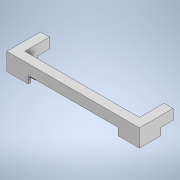
# Autodesk Inventor part: Glass ConnectorV2
Saved by Autodesk Inventor 2022 (Build 260153000, 153)
## iProperties
Created: 2022-05-30
Part Number: Glass ConnectorV2
Material: Generic
Document SubType Name: Modeling
Designer: abdoo
Density: 1 g/cm^3
Appearance: Default
Author: abdoo
Autodesk Inventor part; units mm, degrees
ref_plane "YZ Plane" through (0, 0, 0) normal (1, 0, 0) x (0, 1, 0)
ref_plane "XZ Plane" through (0, 0, 0) normal (0, 1, 0) x (-1, 0, 0)
ref_plane "XY Plane" through (0, 0, 0) normal (0, 0, 1) x (1, 0, 0)
sketch "Sketch1" plane through (0, 0, 0) normal (0, 1, 0) x (-1, 0, 0)
  line L0 (0, 0) -> (3.15, 0)
  line L1 (3.15, 0) -> (3.15, -20)
  line L2 (3.15, -20) -> (0, -20)
  line L3 (0, -20) -> (0, 0)
  line L4 (0, 0) -> (20, 0)
  line L5 (20, 0) -> (20, -3.15)
  line L6 (20, -3.15) -> (0, -3.15)
  line L7 (0, -3.15) -> (0, 0)
  line L8 (-1.5, 1.5) -> (4.65, 1.5)
  line L9 (4.65, 1.5) -> (4.65, -21.5)
  line L10 (4.65, -21.5) -> (-1.5, -21.5)
  line L11 (-1.5, -21.5) -> (-1.5, 1.5)
  line L12 (21.5, 1.5) -> (-1.5, 1.5)
  line L13 (-1.5, 1.5) -> (-1.5, -4.65)
  line L14 (-1.5, -4.65) -> (21.5, -4.65)
  line L15 (21.5, -4.65) -> (21.5, 1.5)
  line L16 (3.15, -20) -> (3.15, -21.5)
  line L17 (0, -20) -> (0, -21.5)
  line L18 (20, 0) -> (21.5, 0)
  line L19 (20, -3.15) -> (21.5, -3.15)
  line L20 (0, 0) -> (87.6, 0)
  line L21 (87.6, 0) -> (87.6, -3.15)
  line L22 (87.6, -3.15) -> (0, -3.15)
  line L23 (0, -3.15) -> (0, 0)
  line L24 (87.6, 0) -> (89.1, 0)
  line L25 (89.1, 0) -> (89.1, -21.5)
  line L26 (89.1, -21.5) -> (87.6, -21.5)
  line L27 (87.6, -21.5) -> (87.6, 0)
  line L28 (89.1, 0) -> (69.1, 0)
  line L29 (69.1, 0) -> (69.1, 1.5)
  line L30 (69.1, 1.5) -> (89.1, 1.5)
  line L31 (89.1, 1.5) -> (89.1, 0)
  line L32 (87.6, -3.15) -> (84.45, -3.15)
  line L33 (84.45, -3.15) -> (84.45, -21.5)
  line L34 (84.45, -21.5) -> (87.6, -21.5)
  line L35 (87.6, -21.5) -> (87.6, -3.15)
  line L36 (84.45, -3.15) -> (82.95, -3.15)
  line L37 (82.95, -3.15) -> (82.95, -21.5)
  line L38 (82.95, -21.5) -> (84.45, -21.5)
  line L39 (84.45, -21.5) -> (84.45, -3.15)
  line L40 (82.95, -3.15) -> (69.1, -3.15)
  line L41 (69.1, -3.15) -> (69.1, -4.65)
  line L42 (69.1, -4.65) -> (82.95, -4.65)
  line L43 (82.95, -4.65) -> (82.95, -3.15)
  line L44 (69.1, -4.65) -> (21.5, -4.65)
  line L45 (21.5, -4.65) -> (21.5, -3.15)
  line L46 (21.5, -3.15) -> (69.1, -3.15)
  line L47 (69.1, -3.15) -> (69.1, -4.65)
  line L48 (69.1, 1.5) -> (21.5, 1.5)
  line L49 (21.5, 1.5) -> (21.5, 0)
  line L50 (21.5, 0) -> (69.1, 0)
  line L51 (69.1, 0) -> (69.1, 1.5)
  point P0 (3.15, -3.15)
  point P1 (4.65, -4.65)
  point P2 (4.65, 1.5)
  point P3 (69.1, 0)
  point P4 (84.45, -3.15)
  point P5 (69.1, -3.15)
  point P6 (21.5, -4.65)
  point P7 (21.5, -3.15)
  dimension "d0" = 3.15
  dimension "d1" = 3.15
  dimension "d2" = 20
  dimension "d3" = 20
  dimension "d4" = 1.5
  dimension "d5" = 1.5
  dimension "d16" = 87.6
  dimension "d17" = 0
  dimension "d18" = 0
  dimension "d19" = 20
  dimension "d20" = 1.5
  dimension "d21" = 3.15
  dimension "d22" = 0
  dimension "d23" = 0
  dimension "d24" = 0
  dimension "d25" = 0
  dimension "d26" = 1.5
  dimension "d27" = 1.5
  constraints: 104 end point, 24 parallel, 16 perpendicular, 10 horizontal, 4 point on line, 6 other
  measures "d0" distance between parallel lines of L4 L6
  measures "d1" distance between parallel lines of L3 L1
  measures "d2" distance of L2.end L0.start
  measures "d3" distance of L0.start L4.end
  measures "d4" distance between parallel lines of L3 L11
  measures "d5" distance between parallel lines of L4 L12
  measures "d16" distance of L0.start L20.end
  measures "d17" distance between parallel lines of L10 L26
  measures "d18" distance between parallel lines of L12 L30
  measures "d19" distance of L29.end L30.end
  measures "d20" distance between parallel lines of L35 L25
  measures "d21" distance of L33.end L34.end
  measures "d22" distance between parallel lines of L6 L22
  measures "d23" distance between parallel lines of L26 L38
  measures "d24" distance between parallel lines of L38 L34
  measures "d25" distance between parallel lines of L29 L41
  measures "d26" distance between parallel lines of L33 L37
  measures "d27" distance between parallel lines of L22 L42
extrude "Extrusion1" add sketch "Sketch1" along normal blind 5 contours L3 L14 L11 L8 L9 L4 L0 | L6 L9 L14 L1 | L9 L12 L15 L18 L4 | L3 L17 L10 L11 L14 | L14 L9 L10 L16 L1 | L6 L19 L15 L14 L9 | L15 L48 L29 L20 | L15 L22 L41 L44 | L29 L30 L31 L24 L20 | L41 L22 L37 L42 | L24 L25 L26 L27 L21 | L37 L22 L33 L38
sketch "Sketch2" plane through (0, 5, 0) normal (0, 1, 0) x (1, 0, 0)
  line L0 (-3.15, 3.15) -> (-3.15, 21.5) projected
  line L1 (-3.15, 21.5) -> (-4.65, 21.5) projected
  line L2 (-4.65, 21.5) -> (-4.65, 4.65) projected
  line L3 (1.5, -1.5) -> (1.5, 21.5) projected
  line L4 (1.5, 21.5) -> (0, 21.5) projected
  line L5 (0, 21.5) -> (0, 0) projected
  line L6 (0, 0) -> (-21.5, 0) projected
  line L7 (-21.5, 0) -> (-21.5, 3)
  line L8 (-3.15, 3.15) -> (-3.15, 21.5) projected
  line L9 (-3.15, 21.5) -> (0, 21.5)
  line L10 (-89.1, 21.5) -> (-89.1, -1.5) projected
  line L11 (-82.95, 4.65) -> (-82.95, 21.5) projected
  line L12 (-89.1, -1.5) -> (-68.78, -1.5) projected
  line L13 (-68.78, 4.5) -> (-82.95, 4.5) projected
  line L14 (-87.6, 21.5) -> (-89.1, 21.5) projected
  line L15 (-89.1, 21.5) -> (-82.95, 21.5)
  line L16 (-82.95, 21.5) -> (-82.95, -1.5)
  line L17 (-82.95, -1.5) -> (-89.1, -1.5)
  line L18 (-89.1, -1.5) -> (-89.1, 21.5)
  line L19 (-68.78, -1.5) -> (-82.95, -1.5)
  line L20 (-82.95, -1.5) -> (-82.95, 4.65)
  line L21 (-82.95, 4.65) -> (-68.78, 4.65)
  line L22 (-68.78, 4.65) -> (-68.78, -1.5)
  line L23 (0, 0) -> (-87.6, 0) projected
  line L24 (-87.6, 0) -> (-87.6, 21.5) projected
  line L25 (-87.6, 21.5) -> (-89.1, 21.5) projected
  line L26 (-89.1, 21.5) -> (-89.1, -1.5) projected
  line L27 (-89.1, -1.5) -> (1.5, -1.5) projected
  line L28 (-84.45, 3.15) -> (-3.15, 3.15) projected
  line L29 (-4.65, 4.65) -> (-82.95, 4.65) projected
  line L30 (-82.95, 4.65) -> (-82.95, 21.5) projected
  line L31 (-82.95, 21.5) -> (-84.45, 21.5) projected
  line L32 (-84.45, 21.5) -> (-84.45, 3.15) projected
  point P0 (-82.95, 4.65)
  point P1 (-68.78, 4.65)
  dimension "d31" = 0
  constraints: 20 end point, 4 parallel, 4 perpendicular, 2 horizontal, 1 point on line, 1 other
  measures "d31" distance between parallel lines of L20 L16
extrude "Extrusion2" add sketch "Sketch2" along normal blind 2
sketch "Sketch3" plane through (0, 0, 0) normal (0, -1, 0) x (1, 0, 0)
  line L0 (-4.65, -21.5) -> (-4.65, -4.65) projected
  line L1 (-3.15, -21.5) -> (-4.65, -21.5) projected
  line L2 (-3.15, -3.15) -> (-3.15, -21.5) projected
  line L3 (0, -21.5) -> (0, 0) projected
  line L4 (1.5, -21.5) -> (0, -21.5) projected
  line L5 (1.5, 1.5) -> (1.5, -21.5) projected
  line L6 (-21.5, -3) -> (-3.15, -3) projected
  line L7 (-4.65, -21.5) -> (-4.65, -4.65) projected
  line L8 (-3.15, -3.15) -> (-4.65, -3.15)
  line L9 (-4.65, -3.15) -> (-4.65, -13.15)
  line L10 (-4.65, -13.15) -> (-3.15, -13.15)
  line L11 (-3.15, -13.15) -> (-3.15, -3.15)
  line L12 (-3.15, -3.15) -> (-3.15, -21.5) projected
  line L13 (-3.15, -3.15) -> (-13.15, -3.15)
  line L14 (-13.15, -3.15) -> (-13.15, -4.65)
  line L15 (-13.15, -4.65) -> (-3.15, -4.65)
  line L16 (-3.15, -4.65) -> (-3.15, -3.15)
  line L17 (-21.5, 1.5) -> (1.5, 1.5) projected
  line L18 (0, -21.5) -> (0, 0) projected
  line L19 (1.5, 1.5) -> (0, 1.5)
  line L20 (0, 1.5) -> (0, -13.15)
  line L21 (0, -13.15) -> (1.5, -13.15)
  line L22 (1.5, -13.15) -> (1.5, 1.5)
  line L23 (1.5, 1.5) -> (-13.15, 1.5)
  line L24 (-13.15, 1.5) -> (-13.15, 0)
  line L25 (-13.15, 0) -> (1.5, 0)
  line L26 (1.5, 0) -> (1.5, 1.5)
  line L27 (-89.1, -21.5) -> (-89.1, 1.5) projected
  line L28 (0, 0) -> (-87.6, 0) projected
  line L29 (-89.1, 1.5) -> (-74.45, 1.5)
  line L30 (-74.45, 1.5) -> (-74.45, 0)
  line L31 (-74.45, 0) -> (-89.1, 0)
  line L32 (-89.1, 0) -> (-89.1, 1.5)
  line L33 (-89.1, 1.5) -> (-68.78, 1.5) projected
  line L34 (-89.1, 1.5) -> (-87.6, 1.5)
  line L35 (-87.6, 1.5) -> (-87.6, -13.15)
  line L36 (-87.6, -13.15) -> (-89.1, -13.15)
  line L37 (-89.1, -13.15) -> (-89.1, 1.5)
  line L38 (-84.45, -21.5) -> (-84.45, -3.15) projected
  line L39 (-74.45, -3.15) -> (-84.45, -3.15)
  line L40 (-84.45, -3.15) -> (-84.45, -4.65)
  line L41 (-84.45, -4.65) -> (-74.45, -4.65)
  line L42 (-74.45, -4.65) -> (-74.45, -3.15)
  line L43 (-84.45, -3.15) -> (-3.15, -3.15) projected
  line L44 (-82.95, -4.65) -> (-82.95, -21.5) projected
  line L45 (-84.45, -3.15) -> (-82.95, -3.15)
  line L46 (-82.95, -3.15) -> (-82.95, -13.075)
  line L47 (-82.95, -13.075) -> (-84.45, -13.075)
  line L48 (-84.45, -13.075) -> (-84.45, -3.15)
  line L49 (0, 0) -> (-87.6, 0) projected
  line L50 (-89.1, 1.5) -> (1.5, 1.5) projected
  line L51 (-89.1, -21.5) -> (-89.1, 1.5) projected
  line L52 (-87.6, -21.5) -> (-89.1, -21.5) projected
  line L53 (-87.6, 0) -> (-87.6, -21.5) projected
  line L54 (-84.45, -3.15) -> (-3.15, -3.15) projected
  line L55 (-84.45, -21.5) -> (-84.45, -3.15) projected
  line L56 (-82.95, -21.5) -> (-84.45, -21.5) projected
  line L57 (-82.95, -4.65) -> (-82.95, -21.5) projected
  line L58 (-4.65, -4.65) -> (-82.95, -4.65) projected
  point P0 (-3.15, -13.15)
  point P1 (-68.78, 0)
  point P2 (-68.78, -3)
  point P3 (1.5, 0)
  point P4 (-3.15, -4.65)
  point P5 (-4.65, -4.65)
  point P6 (-13, -3)
  point P7 (-4.65, -4.65)
  dimension "d10" = 10
  dimension "d11" = 10
  dimension "d12" = 14.65
  dimension "d13" = 14.65
  dimension "d28" = 14.65
  dimension "d29" = 14.65
  dimension "d30" = 10
  dimension "d32" = 0
  dimension "d33" = 0
  constraints: 64 end point, 16 parallel, 8 horizontal, 8 perpendicular, 4 point on line, 1 midpoint, 2 other
  measures "d10" distance of L8.end L9.end
  measures "d11" distance of L14.end L15.end
  measures "d12" distance of L24.end L25.end
  measures "d13" distance of L19.end L20.end
  measures "d28" distance of L27.end L29.end
  measures "d29" distance of L34.end L35.end
  measures "d30" distance of L40.end L41.end
  measures "d32" vertical extent of L39
  measures "d33" distance between parallel lines of L58 L41
extrude "Extrusion3" add sketch "Sketch3" along normal blind 5 contours L0 L15 L2 L10 | L15 L14 L13 L9 | L9 L8 L2 L15 | L41 L46 L39 L42 | L44 L47 L38 L41 | L41 L38 L39 L46 | L3 L25 L5 L21 | L25 L24 L17 L20 | L20 L17 L5 L25 | L28 L35 L29 L30 | L35 L36 L27 L31 | L31 L27 L29 L35
body "Solid1"
